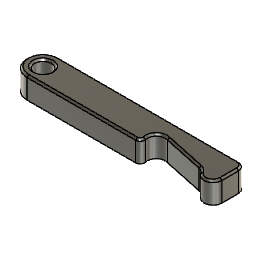
SPIDER PROJECT 1 v2 (Autodesk Fusion 360 design; units mm, degrees)
Autodesk Fusion 360 part; units mm, degrees
note: some values were not read from the file. Set by a fixed rule: which sketch regions a step uses.
sketch "Sketch1" plane through (0, 0, 0) normal (0, 0, 1) x (1, 0, 0)
  line L0 (0, 0) -> (61.1655, 0)
  line L1 (0, 18) -> (101, 18)
  arc A0 (0, 18) -> (0, 0) centre (0, 9) ccw
  line L2 (105, 14) -> (105, 4.6244)
  arc A1 (105, 14) -> (101, 18) centre (101, 14) ccw
  arc A2 (61.1655, 0) -> (63.5932, 3.0968) centre (61.1655, 2.5) ccw
  circle A3 centre (0, 9) radius 4.75
  arc A4 (95.7497, 1.991) -> (105, 4.6244) centre (100, 4.6244) ccw
  arc A5 (70.039, 9.0307) -> (63.5932, 3.0968) centre (68.4487, 4.2904) ccw
  line L3 (70.039, 9.0307) -> (92.539, 4.2482)
  arc A6 (95.7497, 1.991) -> (92.539, 4.2482) centre (91.4995, -0.6425) ccw
  point P0 (95.465, 6.73)
  dimension "d1" = 4
  dimension "d4" = 2.5
  dimension "d6" = 9.5
  dimension "d17" = 5
  dimension "d23" = 5
  dimension "d28" = 5
  dimension "d40" = 101
  dimension "d54" = 5
  dimension "d55" = 12
  dimension "d56" = 22.5
  dimension "d57" = 2.5
  dimension "d58" = 5
  dimension "d59" = 12
  dimension "d60" = 5
  dimension "d61" = 18
  constraint coincident L0.start A0.end
  constraint horizontal L0
  constraint horizontal L1
  constraint tangent L1 A0
  constraint perpendicular L1 L2
  constraint tangent L1 A1
  constraint tangent L2 A1
  constraint tangent L0 A2
  constraint concentric A0 A3
  constraint tangent L2 A4
  constraint coincident P0 A4
  constraint tangent A2 A5
  constraint tangent L3 A6
  constraint tangent A4 A6
  measures "d1" radius of A1
  measures "d4" radius of A2
  measures "d6" diameter of A3
  measures "d17" radius of A4
  measures "d23" radius of A5
  measures "d28" radius of A4
  measures "d40" distance of L1.start L1.end
  measures "d54" radius of A6
  measures "d55" angle of L0 L3
  measures "d56" horizontal distance of A5.start L3.end
  measures "d57" radius of A2
  measures "d58" radius of A5
  measures "d59" angle of L0 L3
  measures "d60" radius of A6
  measures "d61" distance of L0.start L1.start
extrude "Extrude1" add sketch "Sketch1" along normal blind 12
sketch "Sketch6" plane through (0, 0, 0) normal (0, 0, 1) x (1, 0, 0)
sketch "Sketch7" plane through (0, 0, 0) normal (0, 0, 1) x (1, 0, 0)
chamfer "Chamfer1" distance 1 angle 45 1 faces at (87.8593, 10.4263, 12)
sketch "Sketch4" plane through (0, 0, 0) normal (0, 0, 1) x (1, 0, 0)
  line L0 (69.1004, 11.8979) -> (91.6004, 16.6804)
  line L1 (64.1453, 0) -> (0, 0)
  arc A0 (69.1004, 11.8979) -> (66.1436, 4.0024) centre (70.14, 7.0072) ccw
  arc A1 (96.32, 8.4047) -> (91.6004, 16.6804) centre (92.64, 11.7896) ccw
  arc A2 (96.32, 8.4047) -> (105, 5.0198) centre (100, 5.0198) ccw
  arc A3 (105, 14) -> (101, 18) centre (101, 14) ccw
  line L2 (101, 18) -> (0, 18)
  circle A4 centre (0, 9) radius 4.75
  dimension "d44" = 12
  dimension "d45" = 22.5
  dimension "d46" = 5
  dimension "d47" = 5
  dimension "d48" = 5
  dimension "d49" = 4
  dimension "d50" = 101
  dimension "d51" = 18
  dimension "d52" = 9.5
  measures "d44" angle of L0 L1
  measures "d45" horizontal distance of L0.start L0.end
  measures "d46" radius of A0
  measures "d47" radius of A1
  measures "d48" radius of A2
  measures "d49" radius of A3
  measures "d50" distance of A3.end L2.end
  measures "d51" distance of L2.end L1.end
  measures "d52" diameter of A4
sketch "Sketch5" plane through (0, 0, 12) normal (0, 0, 1) x (-1, 0, 0)
  circle A0 centre (0, -9) radius 4.75
  arc A1 (-96.32, -8.4047) -> (-105, -5.0198) centre (-100, -5.0198) ccw
  line L0 (-105, -5.0198) -> (-105, -14)
  arc A2 (-105, -14) -> (-101, -18) centre (-101, -14) ccw
  arc A3 (0, -18) -> (0, 0) centre (0, -9) ccw
  line L1 (0, 0) -> (-64.1453, 0)
  arc A4 (-64.1453, 0) -> (-66.1436, -4.0024) centre (-64.1453, -2.5) ccw
  arc A5 (-69.1004, -11.8979) -> (-66.1436, -4.0024) centre (-70.14, -7.0072) ccw
  line L2 (-69.1004, -11.8979) -> (-91.6004, -16.6804)
  arc A6 (-96.32, -8.4047) -> (-91.6004, -16.6804) centre (-92.64, -11.7896) ccw
